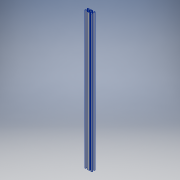
# Autodesk Inventor part: Profile vertical 20x40x750
Saved by Autodesk Inventor 2017 (Build 210142000, 142)
## iProperties
Company: FABLAB Frenchmakers
Part Number: Profile vertical 20x40x750
Material: Aluminium
Document SubType Name: Modeling
Designer: FABLAB Frenchmakers
Density: 2.7 g/cm^3
Appearance: Aluminium - Plat(2)
Mass: 580.495 g
Surface Area: 2454.41 cm^2
Volume: 214.998 cm^3
Stock Number: 1420-01-01
Project: 1420 Vauban 3D XL
Autodesk Inventor part; units mm, degrees
ref_plane "YZ Plane" through (0, 0, 0) normal (1, 0, 0) x (0, 1, 0)
ref_plane "XZ Plane" through (0, 0, 0) normal (0, 1, 0) x (-1, 0, 0)
ref_plane "XY Plane" through (0, 0, 0) normal (0, 0, 1) x (1, 0, 0)
sketch "Esquisse1" plane through (0, 0, 0) normal (0, 0, 1) x (1, 0, 0)
  line L0 (-20, -8.5) -> (-20, -3.7)
  arc A0 (-20, -8.5) -> (-18.5, -10) centre (-18.5, -8.5) ccw
  line L1 (-13.7, -10) -> (-18.5, -10)
  arc A1 (-13.7, -10) -> (-13.5, -9.8) centre (-13.7, -9.8) ccw
  line L2 (-13.5, -9.5) -> (-13.5, -9.8)
  line L3 (-13.2, -9.5) -> (-13.5, -9.5)
  arc A2 (-13.2, -9.5) -> (-13, -9.3) centre (-13.2, -9.3) ccw
  line L4 (-13, -9) -> (-13, -9.3)
  arc A3 (-13, -9) -> (-13.5, -8.5) centre (-13.5, -9) ccw
  line L5 (-15.5, -8.5) -> (-13.5, -8.5)
  arc A4 (-16, -8) -> (-15.5, -8.5) centre (-15.5, -8) ccw
  line L6 (-16, -7.2678) -> (-16, -8)
  arc A5 (-15.8536, -6.9142) -> (-16, -7.2678) centre (-15.5, -7.2678) ccw
  line L7 (-13.5858, -4.6464) -> (-15.8536, -6.9142)
  arc A6 (-13.2322, -4.5) -> (-13.5858, -4.6464) centre (-13.2322, -5) ccw
  line L8 (-10.9536, -4.5) -> (-13.2322, -4.5)
  arc A7 (-10.9536, -4.5) -> (-10.8536, -4.4732) centre (-10.9536, -4.3) ccw
  line L9 (-10.1, -4.0381) -> (-10.8536, -4.4732)
  arc A8 (-9.9, -4.0381) -> (-10.1, -4.0381) centre (-10, -4.2113) ccw
  line L10 (-9.1464, -4.4732) -> (-9.9, -4.0381)
  arc A9 (-9.1464, -4.4732) -> (-9.0464, -4.5) centre (-9.0464, -4.3) ccw
  line L11 (-6.7678, -4.5) -> (-9.0464, -4.5)
  arc A10 (-6.4142, -4.6464) -> (-6.7678, -4.5) centre (-6.7678, -5) ccw
  line L12 (-4.1464, -6.9142) -> (-6.4142, -4.6464)
  arc A11 (-4, -7.2678) -> (-4.1464, -6.9142) centre (-4.5, -7.2678) ccw
  line L13 (-4, -8) -> (-4, -7.2678)
  arc A12 (-4.5, -8.5) -> (-4, -8) centre (-4.5, -8) ccw
  line L14 (-6.5, -8.5) -> (-4.5, -8.5)
  arc A13 (-6.5, -8.5) -> (-7, -9) centre (-6.5, -9) ccw
  line L15 (-7, -9.3) -> (-7, -9)
  arc A14 (-7, -9.3) -> (-6.8, -9.5) centre (-6.8, -9.3) ccw
  line L16 (-6.5, -9.5) -> (-6.8, -9.5)
  line L17 (-6.5, -9.8) -> (-6.5, -9.5)
  arc A15 (-6.5, -9.8) -> (-6.3, -10) centre (-6.3, -9.8) ccw
  line L18 (6.3, -10) -> (-6.3, -10)
  arc A16 (6.3, -10) -> (6.5, -9.8) centre (6.3, -9.8) ccw
  line L19 (6.5, -9.5) -> (6.5, -9.8)
  line L20 (6.8, -9.5) -> (6.5, -9.5)
  arc A17 (6.8, -9.5) -> (7, -9.3) centre (6.8, -9.3) ccw
  line L21 (7, -9) -> (7, -9.3)
  arc A18 (7, -9) -> (6.5, -8.5) centre (6.5, -9) ccw
  line L22 (4.5, -8.5) -> (6.5, -8.5)
  arc A19 (4, -8) -> (4.5, -8.5) centre (4.5, -8) ccw
  line L23 (4, -7.2678) -> (4, -8)
  arc A20 (4.1464, -6.9142) -> (4, -7.2678) centre (4.5, -7.2678) ccw
  line L24 (6.4142, -4.6464) -> (4.1464, -6.9142)
  arc A21 (6.7678, -4.5) -> (6.4142, -4.6464) centre (6.7678, -5) ccw
  line L25 (9.0464, -4.5) -> (6.7678, -4.5)
  arc A22 (9.0464, -4.5) -> (9.1464, -4.4732) centre (9.0464, -4.3) ccw
  line L26 (9.9, -4.0381) -> (9.1464, -4.4732)
  arc A23 (10.1, -4.0381) -> (9.9, -4.0381) centre (10, -4.2113) ccw
  line L27 (10.8536, -4.4732) -> (10.1, -4.0381)
  arc A24 (10.8536, -4.4732) -> (10.9536, -4.5) centre (10.9536, -4.3) ccw
  line L28 (13.2322, -4.5) -> (10.9536, -4.5)
  arc A25 (13.5858, -4.6464) -> (13.2322, -4.5) centre (13.2322, -5) ccw
  line L29 (15.8536, -6.9142) -> (13.5858, -4.6464)
  arc A26 (16, -7.2678) -> (15.8536, -6.9142) centre (15.5, -7.2678) ccw
  line L30 (16, -8) -> (16, -7.2678)
  arc A27 (15.5, -8.5) -> (16, -8) centre (15.5, -8) ccw
  line L31 (13.5, -8.5) -> (15.5, -8.5)
  arc A28 (13.5, -8.5) -> (13, -9) centre (13.5, -9) ccw
  line L32 (13, -9.3) -> (13, -9)
  arc A29 (13, -9.3) -> (13.2, -9.5) centre (13.2, -9.3) ccw
  line L33 (13.5, -9.5) -> (13.2, -9.5)
  line L34 (13.5, -9.8) -> (13.5, -9.5)
  arc A30 (13.5, -9.8) -> (13.7, -10) centre (13.7, -9.8) ccw
  line L35 (18.5, -10) -> (13.7, -10)
  arc A31 (18.5, -10) -> (20, -8.5) centre (18.5, -8.5) ccw
  line L36 (20, -3.7) -> (20, -8.5)
  arc A32 (20, -3.7) -> (19.8, -3.5) centre (19.8, -3.7) ccw
  line L37 (19.5, -3.5) -> (19.8, -3.5)
  line L38 (19.5, -3.2) -> (19.5, -3.5)
  arc A33 (19.5, -3.2) -> (19.3, -3) centre (19.3, -3.2) ccw
  line L39 (19, -3) -> (19.3, -3)
  arc A34 (19, -3) -> (18.5, -3.5) centre (19, -3.5) ccw
  line L40 (18.5, -5.5) -> (18.5, -3.5)
  arc A35 (18, -6) -> (18.5, -5.5) centre (18, -5.5) ccw
  line L41 (17.2678, -6) -> (18, -6)
  arc A36 (16.9142, -5.8536) -> (17.2678, -6) centre (17.2678, -5.5) ccw
  line L42 (14.6464, -3.5858) -> (16.9142, -5.8536)
  arc A37 (14.5, -3.2322) -> (14.6464, -3.5858) centre (15, -3.2322) ccw
  line L43 (14.5, -0.9536) -> (14.5, -3.2322)
  arc A38 (14.5, -0.9536) -> (14.4732, -0.8536) centre (14.3, -0.9536) ccw
  line L44 (14.0381, -0.1) -> (14.4732, -0.8536)
  arc A39 (14.0381, 0.1) -> (14.0381, -0.1) centre (14.2113, 0) ccw
  line L45 (14.4732, 0.8536) -> (14.0381, 0.1)
  arc A40 (14.4732, 0.8536) -> (14.5, 0.9536) centre (14.3, 0.9536) ccw
  line L46 (14.5, 3.2322) -> (14.5, 0.9536)
  arc A41 (14.6464, 3.5858) -> (14.5, 3.2322) centre (15, 3.2322) ccw
  line L47 (16.9142, 5.8536) -> (14.6464, 3.5858)
  arc A42 (17.2678, 6) -> (16.9142, 5.8536) centre (17.2678, 5.5) ccw
  line L48 (18, 6) -> (17.2678, 6)
  arc A43 (18.5, 5.5) -> (18, 6) centre (18, 5.5) ccw
  line L49 (18.5, 3.5) -> (18.5, 5.5)
  arc A44 (18.5, 3.5) -> (19, 3) centre (19, 3.5) ccw
  line L50 (19.3, 3) -> (19, 3)
  arc A45 (19.3, 3) -> (19.5, 3.2) centre (19.3, 3.2) ccw
  line L51 (19.5, 3.5) -> (19.5, 3.2)
  line L52 (19.8, 3.5) -> (19.5, 3.5)
  arc A46 (19.8, 3.5) -> (20, 3.7) centre (19.8, 3.7) ccw
  line L53 (20, 8.5) -> (20, 3.7)
  arc A47 (20, 8.5) -> (18.5, 10) centre (18.5, 8.5) ccw
  line L54 (13.7, 10) -> (18.5, 10)
  arc A48 (13.7, 10) -> (13.5, 9.8) centre (13.7, 9.8) ccw
  line L55 (13.5, 9.5) -> (13.5, 9.8)
  line L56 (13.2, 9.5) -> (13.5, 9.5)
  arc A49 (13.2, 9.5) -> (13, 9.3) centre (13.2, 9.3) ccw
  line L57 (13, 9) -> (13, 9.3)
  arc A50 (13, 9) -> (13.5, 8.5) centre (13.5, 9) ccw
  line L58 (15.5, 8.5) -> (13.5, 8.5)
  arc A51 (16, 8) -> (15.5, 8.5) centre (15.5, 8) ccw
  line L59 (16, 7.2678) -> (16, 8)
  arc A52 (15.8536, 6.9142) -> (16, 7.2678) centre (15.5, 7.2678) ccw
  line L60 (13.5858, 4.6464) -> (15.8536, 6.9142)
  arc A53 (13.2322, 4.5) -> (13.5858, 4.6464) centre (13.2322, 5) ccw
  line L61 (10.9536, 4.5) -> (13.2322, 4.5)
  arc A54 (10.9536, 4.5) -> (10.8536, 4.4732) centre (10.9536, 4.3) ccw
  line L62 (10.1, 4.0381) -> (10.8536, 4.4732)
  arc A55 (9.9, 4.0381) -> (10.1, 4.0381) centre (10, 4.2113) ccw
  line L63 (9.1464, 4.4732) -> (9.9, 4.0381)
  arc A56 (9.1464, 4.4732) -> (9.0464, 4.5) centre (9.0464, 4.3) ccw
  line L64 (6.7678, 4.5) -> (9.0464, 4.5)
  arc A57 (6.4142, 4.6464) -> (6.7678, 4.5) centre (6.7678, 5) ccw
  line L65 (4.1464, 6.9142) -> (6.4142, 4.6464)
  arc A58 (4, 7.2678) -> (4.1464, 6.9142) centre (4.5, 7.2678) ccw
  line L66 (4, 8) -> (4, 7.2678)
  arc A59 (4.5, 8.5) -> (4, 8) centre (4.5, 8) ccw
  line L67 (6.5, 8.5) -> (4.5, 8.5)
  arc A60 (6.5, 8.5) -> (7, 9) centre (6.5, 9) ccw
  line L68 (7, 9.3) -> (7, 9)
  arc A61 (7, 9.3) -> (6.8, 9.5) centre (6.8, 9.3) ccw
  line L69 (6.5, 9.5) -> (6.8, 9.5)
  line L70 (6.5, 9.8) -> (6.5, 9.5)
  arc A62 (6.5, 9.8) -> (6.3, 10) centre (6.3, 9.8) ccw
  line L71 (-6.3, 10) -> (6.3, 10)
  arc A63 (-6.3, 10) -> (-6.5, 9.8) centre (-6.3, 9.8) ccw
  line L72 (-6.5, 9.5) -> (-6.5, 9.8)
  line L73 (-6.8, 9.5) -> (-6.5, 9.5)
  arc A64 (-6.8, 9.5) -> (-7, 9.3) centre (-6.8, 9.3) ccw
  line L74 (-7, 9) -> (-7, 9.3)
  arc A65 (-7, 9) -> (-6.5, 8.5) centre (-6.5, 9) ccw
  line L75 (-4.5, 8.5) -> (-6.5, 8.5)
  arc A66 (-4, 8) -> (-4.5, 8.5) centre (-4.5, 8) ccw
  line L76 (-4, 7.2678) -> (-4, 8)
  arc A67 (-4.1464, 6.9142) -> (-4, 7.2678) centre (-4.5, 7.2678) ccw
  line L77 (-6.4142, 4.6464) -> (-4.1464, 6.9142)
  arc A68 (-6.7678, 4.5) -> (-6.4142, 4.6464) centre (-6.7678, 5) ccw
  line L78 (-9.0464, 4.5) -> (-6.7678, 4.5)
  arc A69 (-9.0464, 4.5) -> (-9.1464, 4.4732) centre (-9.0464, 4.3) ccw
  line L79 (-9.9, 4.0381) -> (-9.1464, 4.4732)
  arc A70 (-10.1, 4.0381) -> (-9.9, 4.0381) centre (-10, 4.2113) ccw
  line L80 (-10.8536, 4.4732) -> (-10.1, 4.0381)
  arc A71 (-10.8536, 4.4732) -> (-10.9536, 4.5) centre (-10.9536, 4.3) ccw
  line L81 (-13.2322, 4.5) -> (-10.9536, 4.5)
  arc A72 (-13.5858, 4.6464) -> (-13.2322, 4.5) centre (-13.2322, 5) ccw
  line L82 (-15.8536, 6.9142) -> (-13.5858, 4.6464)
  arc A73 (-16, 7.2678) -> (-15.8536, 6.9142) centre (-15.5, 7.2678) ccw
  line L83 (-16, 8) -> (-16, 7.2678)
  arc A74 (-15.5, 8.5) -> (-16, 8) centre (-15.5, 8) ccw
  line L84 (-13.5, 8.5) -> (-15.5, 8.5)
  arc A75 (-13.5, 8.5) -> (-13, 9) centre (-13.5, 9) ccw
  line L85 (-13, 9.3) -> (-13, 9)
  arc A76 (-13, 9.3) -> (-13.2, 9.5) centre (-13.2, 9.3) ccw
  line L86 (-13.5, 9.5) -> (-13.2, 9.5)
  line L87 (-13.5, 9.8) -> (-13.5, 9.5)
  arc A77 (-13.5, 9.8) -> (-13.7, 10) centre (-13.7, 9.8) ccw
  line L88 (-18.5, 10) -> (-13.7, 10)
  arc A78 (-18.5, 10) -> (-20, 8.5) centre (-18.5, 8.5) ccw
  line L89 (-20, 3.7) -> (-20, 8.5)
  arc A79 (-20, 3.7) -> (-19.8, 3.5) centre (-19.8, 3.7) ccw
  line L90 (-19.5, 3.5) -> (-19.8, 3.5)
  line L91 (-19.5, 3.2) -> (-19.5, 3.5)
  arc A80 (-19.5, 3.2) -> (-19.3, 3) centre (-19.3, 3.2) ccw
  line L92 (-19, 3) -> (-19.3, 3)
  arc A81 (-19, 3) -> (-18.5, 3.5) centre (-19, 3.5) ccw
  line L93 (-18.5, 5.5) -> (-18.5, 3.5)
  arc A82 (-18, 6) -> (-18.5, 5.5) centre (-18, 5.5) ccw
  line L94 (-17.2678, 6) -> (-18, 6)
  arc A83 (-16.9142, 5.8536) -> (-17.2678, 6) centre (-17.2678, 5.5) ccw
  line L95 (-14.6464, 3.5858) -> (-16.9142, 5.8536)
  arc A84 (-14.5, 3.2322) -> (-14.6464, 3.5858) centre (-15, 3.2322) ccw
  line L96 (-14.5, 0.9536) -> (-14.5, 3.2322)
  arc A85 (-14.5, 0.9536) -> (-14.4732, 0.8536) centre (-14.3, 0.9536) ccw
  line L97 (-14.0381, 0.1) -> (-14.4732, 0.8536)
  arc A86 (-14.0381, -0.1) -> (-14.0381, 0.1) centre (-14.2113, 0) ccw
  line L98 (-14.4732, -0.8536) -> (-14.0381, -0.1)
  arc A87 (-14.4732, -0.8536) -> (-14.5, -0.9536) centre (-14.3, -0.9536) ccw
  line L99 (-14.5, -3.2322) -> (-14.5, -0.9536)
  arc A88 (-14.6464, -3.5858) -> (-14.5, -3.2322) centre (-15, -3.2322) ccw
  line L100 (-16.9142, -5.8536) -> (-14.6464, -3.5858)
  arc A89 (-17.2678, -6) -> (-16.9142, -5.8536) centre (-17.2678, -5.5) ccw
  line L101 (-18, -6) -> (-17.2678, -6)
  arc A90 (-18.5, -5.5) -> (-18, -6) centre (-18, -5.5) ccw
  line L102 (-18.5, -3.5) -> (-18.5, -5.5)
  arc A91 (-18.5, -3.5) -> (-19, -3) centre (-19, -3.5) ccw
  line L103 (-19.3, -3) -> (-19, -3)
  arc A92 (-19.3, -3) -> (-19.5, -3.2) centre (-19.3, -3.2) ccw
  line L104 (-19.5, -3.5) -> (-19.5, -3.2)
  line L105 (-19.8, -3.5) -> (-19.5, -3.5)
  arc A93 (-19.8, -3.5) -> (-20, -3.7) centre (-19.8, -3.7) ccw
  arc A94 (-2.5, -6.6464) -> (-2.6464, -6.2929) centre (-3, -6.6464) ccw
  line L106 (-2.6464, -6.2929) -> (-5.3536, -3.5858)
  arc A95 (-5.5, -3.2322) -> (-5.3536, -3.5858) centre (-5, -3.2322) ccw
  line L107 (-5.5, -3.2322) -> (-5.5, -0.9536)
  arc A96 (-5.5, -0.9536) -> (-5.5268, -0.8536) centre (-5.7, -0.9536) ccw
  line L108 (-5.5268, -0.8536) -> (-5.9619, -0.1)
  arc A97 (-5.9619, 0.1) -> (-5.9619, -0.1) centre (-5.7887, 0) ccw
  line L109 (-5.9619, 0.1) -> (-5.5268, 0.8536)
  arc A98 (-5.5268, 0.8536) -> (-5.5, 0.9536) centre (-5.7, 0.9536) ccw
  line L110 (-5.5, 0.9536) -> (-5.5, 3.2322)
  arc A99 (-5.3536, 3.5858) -> (-5.5, 3.2322) centre (-5, 3.2322) ccw
  line L111 (-5.3536, 3.5858) -> (-2.6464, 6.2929)
  arc A100 (-2.6464, 6.2929) -> (-2.5, 6.6464) centre (-3, 6.6464) ccw
  line L112 (-2.5, 6.6464) -> (-2.5, 8)
  arc A101 (-2, 8.5) -> (-2.5, 8) centre (-2, 8) ccw
  line L113 (-2, 8.5) -> (2, 8.5)
  arc A102 (2.5, 8) -> (2, 8.5) centre (2, 8) ccw
  line L114 (2.5, 8) -> (2.5, 6.6464)
  arc A103 (2.5, 6.6464) -> (2.6464, 6.2929) centre (3, 6.6464) ccw
  line L115 (2.6464, 6.2929) -> (5.3536, 3.5858)
  arc A104 (5.5, 3.2322) -> (5.3536, 3.5858) centre (5, 3.2322) ccw
  line L116 (5.5, 3.2322) -> (5.5, 0.9536)
  arc A105 (5.5, 0.9536) -> (5.5268, 0.8536) centre (5.7, 0.9536) ccw
  line L117 (5.5268, 0.8536) -> (5.9619, 0.1)
  arc A106 (5.9619, -0.1) -> (5.9619, 0.1) centre (5.7887, 0) ccw
  line L118 (5.9619, -0.1) -> (5.5268, -0.8536)
  arc A107 (5.5268, -0.8536) -> (5.5, -0.9536) centre (5.7, -0.9536) ccw
  line L119 (5.5, -0.9536) -> (5.5, -3.2322)
  arc A108 (5.3536, -3.5858) -> (5.5, -3.2322) centre (5, -3.2322) ccw
  line L120 (5.3536, -3.5858) -> (2.6464, -6.2929)
  arc A109 (2.6464, -6.2929) -> (2.5, -6.6464) centre (3, -6.6464) ccw
  line L121 (2.5, -6.6464) -> (2.5, -8)
  arc A110 (2, -8.5) -> (2.5, -8) centre (2, -8) ccw
  line L122 (2, -8.5) -> (-2, -8.5)
  arc A111 (-2.5, -8) -> (-2, -8.5) centre (-2, -8) ccw
  line L123 (-2.5, -8) -> (-2.5, -6.6464)
  arc A112 (-12.9896, -1.9139) -> (-11.9099, -2.9922) centre (-10, 0) ccw
  line L124 (-12.9896, -1.9139) -> (-12.4453, -1.2582)
  arc A113 (-12.4453, 1.2582) -> (-12.4453, -1.2582) centre (-10, 0) ccw
  line L125 (-12.4453, 1.2582) -> (-12.9896, 1.9139)
  arc A114 (-11.9099, 2.9922) -> (-12.9896, 1.9139) centre (-10, 0) ccw
  line L126 (-11.9099, 2.9922) -> (-11.2582, 2.4453)
  arc A115 (-8.7418, 2.4453) -> (-11.2582, 2.4453) centre (-10, 0) ccw
  line L127 (-8.7418, 2.4453) -> (-8.0901, 2.9922)
  arc A116 (-7.0104, 1.9139) -> (-8.0901, 2.9922) centre (-10, 0) ccw
  line L128 (-7.0104, 1.9139) -> (-7.5547, 1.2582)
  arc A117 (-7.5547, -1.2582) -> (-7.5547, 1.2582) centre (-10, 0) ccw
  line L129 (-7.5547, -1.2582) -> (-7.0104, -1.9139)
  arc A118 (-8.0901, -2.9922) -> (-7.0104, -1.9139) centre (-10, 0) ccw
  line L130 (-8.0901, -2.9922) -> (-8.7418, -2.4453)
  arc A119 (-11.2582, -2.4453) -> (-8.7418, -2.4453) centre (-10, 0) ccw
  line L131 (-11.2582, -2.4453) -> (-11.9099, -2.9922)
  arc A120 (7.0104, -1.9139) -> (8.0901, -2.9922) centre (10, 0) ccw
  line L132 (7.0104, -1.9139) -> (7.5547, -1.2582)
  arc A121 (7.5547, 1.2582) -> (7.5547, -1.2582) centre (10, 0) ccw
  line L133 (7.5547, 1.2582) -> (7.0104, 1.9139)
  arc A122 (8.0901, 2.9922) -> (7.0104, 1.9139) centre (10, 0) ccw
  line L134 (8.0901, 2.9922) -> (8.7418, 2.4453)
  arc A123 (11.2582, 2.4453) -> (8.7418, 2.4453) centre (10, 0) ccw
  line L135 (11.2582, 2.4453) -> (11.9099, 2.9922)
  arc A124 (12.9896, 1.9139) -> (11.9099, 2.9922) centre (10, 0) ccw
  line L136 (12.9896, 1.9139) -> (12.4453, 1.2582)
  arc A125 (12.4453, -1.2582) -> (12.4453, 1.2582) centre (10, 0) ccw
  line L137 (12.4453, -1.2582) -> (12.9896, -1.9139)
  arc A126 (11.9099, -2.9922) -> (12.9896, -1.9139) centre (10, 0) ccw
  line L138 (11.9099, -2.9922) -> (11.2582, -2.4453)
  arc A127 (8.7418, -2.4453) -> (11.2582, -2.4453) centre (10, 0) ccw
  line L139 (8.7418, -2.4453) -> (8.0901, -2.9922)
  line L140 (-10, 0) -> (10, 0) construction
  line L141 (0, -8.5) -> (0, 8.5) construction
  point P0 (0, 0)
  point P1 (-6.3, -10)
  point P2 (0, 0)
  constraints: 284 end point, 256 point on circle, 128 centre point, 4 midpoint, 1 horizontal
extrude "Extrusion1" add sketch "Esquisse1" along normal mid plane 750
